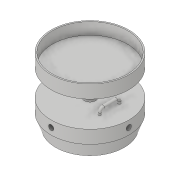
# Autodesk Inventor part: bulkhead v2
Saved by Autodesk Inventor 2019 (Build 230136000, 136)
## iProperties
Created: 2020-10-13
Part Number: bulkhead v2
Material: Generic
Document SubType Name: Sheet Metal
Designer: Nikolas
Density: 1 g/cm^3
Sheet Metal Rule: Default_mm
Appearance: Default
Author: Nikolas
Autodesk Inventor part; units mm, degrees
sketch "Sketch1" plane through (0, 0, 0) normal (0, 0, 1) x (1, 0, 0)
  line L0 (0, 0) -> (2.5, 0)
  line L1 (2.5, 0) -> (2.5, 40)
  line L2 (2.5, 40) -> (7.5, 40)
  line L3 (7.5, 40) -> (7.5, 50)
  line L4 (7.5, 50) -> (8.5, 50)
  line L5 (8.5, 50) -> (8.5, 40)
  line L6 (8.5, 40) -> (59.5, 40)
  line L7 (59.5, 40) -> (59.5, 20)
  line L8 (2.5, 0) -> (52.5, 0)
  line L9 (52.5, 0) -> (59.5, 20)
  line L10 (0, 0) -> (0, 69.9438)
  dimension "d0" = 2.5
  dimension "d1" = 40
  dimension "d2" = 5
  dimension "d3" = 10
  dimension "d4" = 1
  dimension "d5" = 10
  dimension "d6" = 51
  dimension "d7" = 20
  dimension "d8" = 50
  constraints: 22 end point, 4 perpendicular, 3 horizontal, 1 point on line, 1 vertical
  measures "d0" distance of L0.start L0.end
  measures "d1" distance of L0.end L1.end
  measures "d2" distance of L1.end L2.end
  measures "d3" distance of L2.end L3.end
  measures "d4" distance of L3.end L4.end
  measures "d5" distance of L4.end L5.end
  measures "d6" distance of L5.end L6.end
  measures "d7" distance of L6.end L7.end
  measures "d8" distance of L0.end L8.end
revolve "Revolution1" add sketch "Sketch1" angle 360 about axis through (0, 0, 0) along (0, 1, 0)
sketch "Sketch2" plane through (0, 0, 0) normal (1, 0, 0) x (0, 1, 0)
  point P0 (0, 0)
sketch "Sketch3" plane through (0, 0, 0) normal (1, 0, 0) x (0, 1, 0)
  point P0 (0, 0)
ref_plane "Work Plane1" through (59.5, 30, 0) normal (1, 0, 0) x (0, 1, 0)
sketch "Sketch4" plane through (59.5, 30, 0) normal (1, 0, 0) x (0, 1, 0)
  line L0 (-30, 0) -> (0, 0)
  dimension "d10" = 30
  constraints: 2 end point, 1 horizontal
  measures "d10" distance of L0.start L0.end
hole "Hole1" at (59.5, 30, 0) direction (-1, 0, 0) diameter 8 depth 15
thread "Thread1"
ref_plane "Work Plane2" through (0, 30, -59.5) normal (0, 0, 1) x (1, 0, 0)
sketch "Sketch5" plane through (0, 30, -59.5) normal (0, 0, 1) x (1, 0, 0)
  line L0 (0, -30) -> (0, 0)
  dimension "d20" = 30
  constraints: 2 end point, 1 vertical
  measures "d20" distance of L0.start L0.end
hole "Hole2" at (0, 30, -59.5) direction (0, 0, 1) diameter 8 depth 15
thread "Thread2"
ref_plane "Work Plane3" through (-59.5, 30, 0) normal (1, 0, 0) x (0, 1, 0)
sketch "Sketch6" plane through (-59.5, 30, 0) normal (1, 0, 0) x (0, 1, 0)
  line L0 (-30, 0) -> (0, 0)
  dimension "d30" = 30
  constraints: 2 end point, 1 horizontal
  measures "d30" distance of L0.start L0.end
hole "Hole3" at (-59.5, 30, 0) direction (1, 0, 0) diameter 8 depth 15
ref_plane "Work Plane4" through (0, 30, 59.5) normal (0, 0, 1) x (1, 0, 0)
sketch "Sketch7" plane through (0, 30, 59.5) normal (0, 0, 1) x (1, 0, 0)
  line L0 (0, -30) -> (0, 0)
  dimension "d38" = 30
  constraints: 2 end point, 1 vertical
  measures "d38" distance of L0.start L0.end
hole "Hole4" at (0, 30, 59.5) direction (0, 0, -1) diameter 8 depth 15
thread "Thread3"
thread "Thread4"
sketch "Sketch8" plane through (0, 40, 0) normal (0, 1, 0) x (1, 0, 0)
  line L0 (0, 0) -> (30, 0)
  line L1 (30, 0) -> (30, -15)
  circle A0 centre (30, -15) radius 2
  dimension "d50" = 30
  dimension "d51" = 15
  dimension "d52" = 4
  constraints: 4 end point, 1 centre point, 1 coincident, 1 horizontal, 1 perpendicular
  measures "d50" distance of L0.start L0.end
  measures "d51" distance of L0.end L1.end
  measures "d52" diameter of A0
sketch3d "3D Sketch1"
  line L0 (30, 40, 15) -> (30, 43, 15)
  arc A0 (30, 43, 15) -> (30, 48, 10) centre (30, 43, 10) ccw
  line L1 (30, 48, 10) -> (30, 48, -10)
  arc A1 (30, 48, -10) -> (30, 43, -15) centre (30, 43, -10) ccw
  line L2 (30, 43, -15) -> (30, 40, -15)
  dimension "d53" = 5
  dimension "d54" = 5
sweep "Sweep1" add profiles "Sketch8" path "3D Sketch1"
sketch "Sketch9" plane through (0, 40, 0) normal (0, 1, 0) x (1, 0, 0)
  point P0 (0, 0)
sketch "Sketch10" plane through (0, 40, 0) normal (0, 1, 0) x (1, 0, 0)
  point P0 (0, 0)
sketch "Sketch11" plane through (0, 40, 0) normal (0, 1, 0) x (1, 0, 0)
  point P0 (0, 0)
sketch3d "3D Sketch2"
ref_plane "Work Plane5" through (0, 80, 0) normal (0, 0, 1) x (1, 0, 0)
sketch "Sketch12" plane through (0, 80, 0) normal (0, 0, 1) x (1, 0, 0)
  line L0 (0, 0) -> (-59.5, 0)
  line L1 (-59.5, 0) -> (-59.5, 20)
  line L2 (-59.5, 20) -> (-57.5, 20)
  line L3 (-57.5, 20) -> (-57.5, 2)
  line L4 (-57.5, 2) -> (0, 2)
  line L5 (0, 2) -> (0, 0)
  point P0 (0, -80)
  dimension "d57" = 59.5
  dimension "d58" = 20
  dimension "d59" = 2
  dimension "d60" = 18
  constraints: 12 end point, 5 perpendicular, 1 horizontal
  measures "d57" distance of L0.start L0.end
  measures "d58" distance of L0.end L1.end
  measures "d59" distance of L1.end L2.end
  measures "d60" distance of L2.end L3.end
revolve "Revolution2" add sketch "Sketch12" angle 360 about axis through (0, 82, 0) along (0, -1, 0)
equation "\"d54\" = d53"
equation "\"BendRadius\" = Thickness"
equation "\"BendReliefWidth\" = Thickness"
equation "\"BendReliefDepth\" = 0.5 * Thickness"
equation "\"CornerReliefSize\" = 4 * Thickness"
equation "\"MinimumRemnant\" = 2 * Thickness"
equation "\"TransitionRadius\" = BendRadius"
equation "\"JacobiRadiusSize\" = BendRadius"
equation "\"GapSize\" = Thickness"
equation "\"Thickness\" = 0.5"
body "Solid1"
